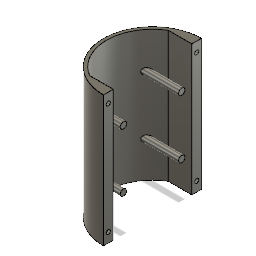
Shell4L v1 (Autodesk Fusion 360 design; units mm, degrees)
Autodesk Fusion 360 part; units mm, degrees
sketch "Sketch1" plane through (0, 0, 0) normal (0, 1, 0) x (1, 0, 0)
  circle A0 centre (0, 0) radius 38.1
  dimension "d1" = 76.2
  constraint coincident A0.centre origin
  measures "d1" diameter of A0
extrude "Extrude1" add sketch "Sketch1" against normal blind 101.6
sketch "Sketch2" plane through (0, 0, 0) normal (0, 1, 0) x (1, 0, 0)
  circle A0 centre (0, 0) radius 35.56
  dimension "d4" = 71.12
  constraint coincident A0.centre origin
  measures "d4" diameter of A0
extrude "Extrude2" cut sketch "Sketch2" against normal blind 154.94
sketch "Sketch3" plane through (0, 0, 0) normal (0, 1, 0) x (1, 0, 0)
  line L0 (0, 38.1) -> (0, -38.1)
  circle A0 centre (0, 0) radius 35.56
  circle A1 centre (0, 0) radius 38.1
  constraint vertical L0
  constraint coincident A0.centre A1.centre
  constraint concentric A0 A1
  constraint coincident L0.start A1
extrude "Extrude3" cut sketch "Sketch3" against normal blind 116.84 contours L0 A0 A1 picked at (3.4943, -37.0034)
sketch "Sketch4" plane through (0, 0, 0) normal (1, 0, 0) x (0, 0, -1)
  line L0 (35.56, -101.6) -> (38.1, -101.6)
  line L1 (38.1, -101.6) -> (38.1, 0)
  line L2 (38.1, 0) -> (35.56, 0)
  line L3 (35.56, 0) -> (35.56, -101.6)
  line L4 (38.1, 0) -> (30.48, 0)
  line L5 (30.48, 0) -> (30.48, -101.6)
  line L6 (30.48, -101.6) -> (38.1, -101.6)
  line L7 (38.1, -101.6) -> (38.1, 0)
  line L8 (-38.1, 0) -> (-30.48, 0)
  line L9 (-30.48, 0) -> (-30.48, -101.6)
  line L10 (-30.48, -101.6) -> (-38.1, -101.6)
  line L11 (-38.1, -101.6) -> (-38.1, 0)
  constraint horizontal L4
  constraint vertical L5
  constraint horizontal L6
  constraint vertical L7
  constraint coincident L1.end L2.start
  constraint horizontal L8
  constraint vertical L9
  constraint horizontal L10
  constraint vertical L11
extrude "Extrude4" add sketch "Sketch4" against normal blind 55.88 contours L3 L4 L5 L6 | L8 L9 L10 L11
sketch "Sketch5" plane through (0, 0, 0) normal (0, 1, 0) x (-1, 0, 0)
  line L0 (0, -30.48) -> (0, -38.1)
  arc A0 (0, -38.1) -> (13.6783, -35.56) centre (0, 0) ccw
  line L1 (13.6783, -35.56) -> (55.88, -35.56)
  line L2 (55.88, -35.56) -> (55.88, -30.48)
  line L3 (55.88, -30.48) -> (22.86, -30.48)
  arc A1 (22.86, -30.48) -> (22.86, 30.48) centre (0, 0) ccw
  line L4 (22.86, 30.48) -> (55.88, 30.48)
  line L5 (55.88, 30.48) -> (55.88, 38.1)
  line L6 (55.88, 38.1) -> (0, 38.1)
  line L7 (0, 38.1) -> (0, 30.48)
  line L8 (0, 30.48) -> (18.3162, 30.48)
  arc A2 (18.3162, -30.48) -> (18.3162, 30.48) centre (0, 0) ccw
  line L9 (18.3162, -30.48) -> (0, -30.48)
  circle A3 centre (0, 0) radius 38.1
  circle A4 centre (0, 0) radius 71.8421
  constraint concentric A0 A3
  constraint concentric A0 A4
extrude "Extrude5" cut sketch "Sketch5" against normal blind 121.92 contours L1 L2 L3 A3 | L4 L5 L6 A3 | A4
sketch "Sketch6" plane through (0, 0, 0) normal (1, 0, 0) x (0, 0, -1)
  line L0 (35.56, -101.6) -> (38.1, -101.6)
  line L1 (38.1, -101.6) -> (38.1, 0)
  line L2 (38.1, 0) -> (30.48, 0)
  line L3 (30.48, 0) -> (30.48, -101.6)
  line L4 (30.48, -101.6) -> (35.56, -101.6)
  line L5 (-30.48, 0) -> (30.48, 0)
  circle A0 centre (22.6462, -28.194) radius 2.5
  circle A1 centre (-22.5658, -28.194) radius 2.5
  circle A2 centre (22.6462, -73.406) radius 2.5
  circle A3 centre (-22.5658, -73.406) radius 2.5
  dimension "d22" = 5
  dimension "d23" = 5
  dimension "d24" = 5
  dimension "d25" = 5
  constraint horizontal L5
  measures "d22" diameter of A0
  measures "d23" diameter of A1
  measures "d24" diameter of A2
  measures "d25" diameter of A3
extrude "Extrude6" add sketch "Sketch6" against normal blind 33.02 contours A0 | A1 | A2 | A3
sketch "Sketch7" plane through (0, 0, 0) normal (0, 1, 0) x (-1, 0, 0)
  arc A0 (0, -38.1) -> (0, 38.1) centre (0, 0) ccw
  line L0 (0, 38.1) -> (0, 30.48)
  line L1 (0, 30.48) -> (18.3162, 30.48)
  arc A1 (18.3162, -30.48) -> (18.3162, 30.48) centre (0, 0) ccw
  line L2 (18.3162, -30.48) -> (0, -30.48)
  line L3 (0, -30.48) -> (0, -38.1)
  circle A2 centre (0, 0) radius 38.1
  circle A3 centre (0, 0) radius 58.6405
  constraint concentric A0 A2
  constraint coincident A0.start A2
  constraint concentric A2 A3
extrude "Extrude7" cut sketch "Sketch7" against normal blind 109.22
sketch "Sketch8" plane through (0, 0, 0) normal (1, 0, 0) x (0, 0, -1)
  circle A0 centre (-22.5658, -28.194) radius 2.5
  circle A1 centre (-22.5658, -28.194) radius 1.625
  line L0 (-38.1, 0) -> (-30.48, 0)
  line L1 (-30.48, -101.6) -> (-38.1, -101.6)
  line L2 (-30.48, -93.98) -> (-38.1, -93.98)
  circle A2 centre (-34.29, -93.98) radius 1.625
  line L3 (-38.1, -7.62) -> (-30.48, -7.62)
  circle A3 centre (-34.29, -7.62) radius 1.625
  dimension "d30" = 3.25
  dimension "d33" = 7.62
  dimension "d34" = 3.25
  dimension "d35" = 7.62
  dimension "d36" = 3.25
  constraint concentric A0 A1
  constraint horizontal L0
  constraint horizontal L1
  constraint midpoint L2 A2.centre
  constraint midpoint L3 A3.centre
  measures "d30" diameter of A1
  measures "d33" distance of L1
  measures "d34" diameter of A2
  measures "d35" distance of L0
  measures "d36" diameter of A3
extrude "Extrude8" cut sketch "Sketch8" against normal blind 4 contours L2 A2 | L2 A2 | L3 A3 | L3 A3
sketch "Sketch9" plane through (0, 0, 0) normal (1, 0, 0) x (0, 0, -1)
  line L0 (35.56, -101.6) -> (38.1, -101.6)
  line L1 (38.1, -101.6) -> (38.1, 0)
  line L2 (38.1, 0) -> (30.48, 0)
  line L3 (30.48, -101.6) -> (35.56, -101.6)
  line L4 (30.48, 0) -> (38.1, 0)
  line L5 (38.1, -101.6) -> (30.48, -101.6)
  circle A0 centre (34.29, -93.98) radius 1.625
  circle A1 centre (34.29, -7.62) radius 1.625
  dimension "d42" = 3.25
  dimension "d43" = 3.25
  constraint horizontal L4
  constraint horizontal L5
  constraint coincident L0.end L1.start
  constraint coincident L2.end L4.start
  measures "d42" diameter of A0
  measures "d43" diameter of A1
extrude "Extrude9" cut sketch "Sketch9" against normal blind 4
